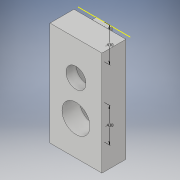
# Autodesk Inventor part: part2
Saved by Autodesk Inventor 2018 (Build 220112000, 112)
## iProperties
Created: 2019-12-04
Part Number: part2
Material: Generic
Document SubType Name: Modeling
Designer: AOFUser
Density: 1 g/cm^3
Appearance: Default
Author: AOFUser
Autodesk Inventor part; units mm, degrees
ref_plane "YZ Plane" through (0, 0, 0) normal (1, 0, 0) x (0, 1, 0)
ref_plane "XZ Plane" through (0, 0, 0) normal (0, 1, 0) x (-1, 0, 0)
ref_plane "XY Plane" through (0, 0, 0) normal (0, 0, 1) x (1, 0, 0)
sketch "Sketch1" plane through (0, 0, 0) normal (0, 1, 0) x (-1, 0, 0)
  line L0 (8.2539, 3.8822) -> (-8.2561, 3.8822)
  line L1 (-8.2561, 3.8822) -> (-8.2561, -3.7378)
  line L2 (-8.2561, -3.7378) -> (8.2539, -3.7378)
  line L3 (8.2539, -3.7378) -> (8.2539, 3.8822)
  line L4 (2.5087, -3.7583) -> (-2.5713, -3.7583)
  line L5 (-2.5713, -3.7583) -> (-2.5713, -5.0283)
  line L6 (-2.5713, -5.0283) -> (2.5087, -5.0283)
  line L7 (2.5087, -5.0283) -> (2.5087, -3.7583)
  point P0 (0, 0)
  dimension "d0" = 16.51
  dimension "d1" = 7.62
  dimension "d2" = 5.08
  dimension "d3" = 1.27
  constraints: 16 end point, 4 parallel, 2 horizontal, 2 perpendicular
  measures "d0" distance of L2.end L1.end
  measures "d1" distance of L1.end L0.end
  measures "d2" distance of L6.end L5.end
  measures "d3" distance of L5.end L4.end
extrude "Extrusion1" add sketch "Sketch1" along normal blind 33.02
sketch "Sketch2" plane through (2.5713, 0, -5.0283) normal (0, 0, -1) x (-1, 0, 0)
  line L0 (10.8253, 33.02) -> (-5.6847, 33.02) projected
  line L1 (2.5703, 33.02) -> (2.5703, 22.098)
  line L2 (2.5713, 0) -> (2.5713, 10.922)
  dimension "d6" = 10.922
  dimension "d7" = 10.922
  constraints: 4 end point, 2 vertical, 1 midpoint
  measures "d6" distance of L1.start L1.end
  measures "d7" distance of L2.start L2.end
sketch "Sketch3" plane through (-8.2539, 0, -3.7378) normal (-1, 0, 0) x (0, 0, 1)
  point P0 (3.7378, 0)
sketch "Sketch4" plane through (-8.2539, 0, 3.8822) normal (0, 0, 1) x (1, 0, 0)
  line L0 (8.2539, 0) -> (8.2539, 10.922)
  line L1 (0, 33.02) -> (16.51, 33.02) projected
  line L2 (8.255, 33.02) -> (8.255, 22.098)
  dimension "d8" = 10.922
  dimension "d9" = 10.922
  constraints: 4 end point, 2 vertical, 1 midpoint
  measures "d8" distance of L0.start L0.end
  measures "d9" distance of L2.start L2.end
hole "Hole1" at (0.0011, 22.098, 3.8822) direction (0, 0, -1) diameter 3.048 end through all counterbore diameter 6.35 counterbore depth 3.302
sketch "Sketch5" plane through (2.5713, 0, -5.0283) normal (0, 0, -1) x (-1, 0, 0)
  point P0 (2.5713, 0)
sketch "Sketch6" plane through (-8.2539, 0, 3.8822) normal (0, 0, 1) x (1, 0, 0)
  line L0 (8.2539, 0) -> (8.2539, 10.9312)
  constraints: 2 end point, 1 vertical
hole "Hole4" at (0, 10.9312, 3.8822) direction (0, 0, -1) diameter 5.08 end through all counterbore diameter 8.89 counterbore depth 5.588
body "Solid1"
